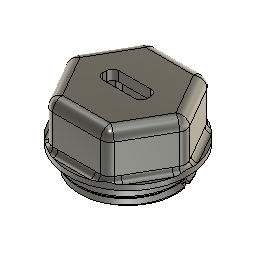
pico_wartel (Autodesk Fusion 360 design; units mm, degrees)
Autodesk Fusion 360 part; units mm, degrees
note: some values were not read from the file. Set by a fixed rule: which sketch regions a step uses.
sketch "Sketch1" plane through (0, 0, 0) normal (0, 0, 1) x (1, 0, 0)
  circle A0 centre (0, 0) radius 10
  constraint coincident A0.centre origin
extrude "Extrude1" add sketch "Sketch1" along normal blind 5
thread "Thread1" "ISO Metric profile 20.0 M20x1.5 6g" major diameter 19.85 minor diameter 18.137 pitch 1.5 angle 60 modelled right hand crest width 0.2154 on face at (9.9876, -0.4985, 3.3333) crest through (9.925, 0, -0.375)
sketch "Sketch2" plane through (0, 0, 5) normal (0, 0, 1) x (-1, 0, 0)
  spline S0 degree 3 poles (5.5723, 8.2131) (4.4831, 8.8876) (3.2736, 9.3446) (0.7674, 9.7621) (-0.5039, 9.7263) (-2.9402, 9.1703) (-4.0834, 8.6632) (-6.0919, 7.248) (-6.9423, 6.3601) (-8.0251, 4.6616) (-8.3649, 3.9377) (-8.8462, 2.4291) (-8.9878, 1.6514) (-9.0271, 0.8652) knots 0 0 0 0 0.384331 0.384331 0.76251 0.76251 1.134533 1.134533 1.5004 1.5004 1.739669 1.739669 1.9762 1.9762 1.9762 1.9762
  arc A0 (-9.0271, 0.8652) -> (-3.7642, -8.2503) centre (0, 0) ccw
  spline S1 degree 3 poles (-3.7642, -8.2503) (-2.7053, -8.7931) (-1.5499, -9.1219) (0.8427, -9.3239) (2.0575, -9.1871) (4.3877, -8.453) (5.4781, -7.8552) (7.3873, -6.2646) (8.1826, -5.2812) (9.1631, -3.4286) (9.4586, -2.6354) (9.8416, -0.9842) (9.9252, -0.1326) (9.8989, 0.7191) knots 0 0 0 0 0.356967 0.356967 0.720082 0.720082 1.089343 1.089343 1.464748 1.464748 1.717242 1.717242 1.972467 1.972467 1.972467 1.972467
  arc A1 (9.8989, 0.7191) -> (5.5723, 8.2131) centre (0, 0) ccw
  circle A2 centre (0, 0) radius 12
  dimension "d3" = 24
  constraint concentric A0 A2
  measures "d3" diameter of A2
extrude "Extrude2" add sketch "Sketch2" along normal blind 1 contours S0 A0 S1 A1 | A2
sketch "Sketch3" plane through (0, 0, 6) normal (0, 0, 1) x (-1, 0, 0)
  circle A0 centre (0, 0) radius 12
  line L0 (-6, -10.3923) -> (6, -10.3923)
  line L1 (6, -10.3923) -> (12, 0)
  line L2 (12, 0) -> (6, 10.3923)
  line L3 (6, 10.3923) -> (-6, 10.3923)
  line L4 (-6, 10.3923) -> (-12, 0)
  line L5 (-12, 0) -> (-6, -10.3923)
  constraint coincident A0.centre origin
  constraint horizontal L0
  constraint coincident A0 L4.end
extrude "Extrude3" add sketch "Sketch3" along normal blind 9 contours L0 L1 L2 L3 L4 L5
sketch "Sketch5" plane through (0, 0, 15) normal (0, 0, 1) x (-1, 0, 0)
  line L0 (-12, 0) -> (-6, -10.3923)
  line L1 (-6, -10.3923) -> (6, -10.3923)
  line L2 (6, -10.3923) -> (12, 0)
  line L3 (12, 0) -> (6, 10.3923)
  line L4 (6, 10.3923) -> (-6, 10.3923)
  line L5 (-6, 10.3923) -> (-12, 0)
  line L6 (-3, 1.625) -> (3.5, 1.625)
  line L7 (4.75, 0.375) -> (4.75, -0.375)
  line L8 (3.5, -1.625) -> (-3, -1.625)
  line L9 (-4.25, -0.375) -> (-4.25, 0.375)
  arc A0 (-3, 1.625) -> (-4.25, 0.375) centre (-3, 0.375) ccw
  arc A1 (-4.25, -0.375) -> (-3, -1.625) centre (-3, -0.375) ccw
  arc A2 (3.5, -1.625) -> (4.75, -0.375) centre (3.5, -0.375) ccw
  arc A3 (4.75, 0.375) -> (3.5, 1.625) centre (3.5, 0.375) ccw
  line L10 (-6, 10.3923) -> (6, -10.3923) construction
  dimension "d40" = 9
  dimension "d41" = 1.25
  dimension "d42" = 3.25
  constraint horizontal L6
  constraint horizontal L8
  constraint vertical L9
  constraint tangent L6 A0
  constraint tangent L9 A0
  constraint tangent L8 A1
  constraint tangent L9 A1
  constraint equal A0 A1
  constraint tangent L7 A2
  constraint tangent L8 A2
  constraint equal A0 A2
  constraint tangent L6 A3
  constraint tangent L7 A3
  constraint equal A0 A3
  constraint coincident L4.end L5.start
  constraint coincident L1.end L2.start
  measures "d40" distance of L7 L9
  measures "d41" radius of A0
  measures "d42" distance of L6 L8
extrude "Extrude5" cut sketch "Sketch5" against normal through all contours L6 L7 L8 L9 A0 A1 A2 A3
sketch "Sketch6" plane through (0, 0, 0) normal (0, 0, -1) x (1, 0, 0)
  line L0 (4.25, 0.375) -> (4.25, -0.375)
  arc A0 (3, -1.625) -> (4.25, -0.375) centre (3, -0.375) ccw
  line L1 (3, -1.625) -> (-3.5, -1.625)
  arc A1 (-4.75, -0.375) -> (-3.5, -1.625) centre (-3.5, -0.375) ccw
  line L2 (-4.75, -0.375) -> (-4.75, 0.375)
  arc A2 (-3.5, 1.625) -> (-4.75, 0.375) centre (-3.5, 0.375) ccw
  line L3 (-3.5, 1.625) -> (3, 1.625)
  arc A3 (4.25, 0.375) -> (3, 1.625) centre (3, 0.375) ccw
  line L4 (-9.25, -1.625) -> (9.25, -1.625)
  line L5 (9.25, -1.625) -> (9.25, -2.875)
  line L6 (9.25, -2.875) -> (-9.25, -2.875)
  line L7 (-9.25, -2.875) -> (-9.25, -1.625)
  line L8 (0, 12.1614) -> (0, -9.8386) construction
  line L9 (-4.75, 0) -> (-4.75, -1.625)
  line L10 (4.25, 0) -> (4.25, -1.625)
  line L11 (5.5, -2.875) -> (-5.5, -2.875)
  line L12 (-5.5, -2.875) -> (-5.5, -4.375)
  line L13 (-5.5, -4.375) -> (5.5, -4.375)
  line L14 (5.5, -4.375) -> (5.5, -2.875)
  line L15 (6.5, -1.625) -> (-6.5, -1.625)
  line L16 (-6.5, -1.625) -> (-6.5, 1.375)
  line L17 (-6.5, 1.375) -> (6.5, 1.375)
  line L18 (6.5, 1.375) -> (6.5, -1.625)
  spline S0 degree 3 poles (-5.2629, 7.3851) (-6.2623, 6.7394) (-7.1248, 5.9032) (-8.4961, 3.9321) (-8.985, 2.8117) (-9.5144, 0.4267) (-9.5419, -0.8166) (-9.119, -3.2653) (-8.6649, -4.4457) (-7.5508, -6.2211) (-7.0116, -6.8737) (-5.7732, -8.031) (-5.0775, -8.5292) (-4.3267, -8.9323) knots 0 0 0 0 0.356967 0.356967 0.720082 0.720082 1.089343 1.089343 1.464748 1.464748 1.717242 1.717242 1.972467 1.972467 1.972467 1.972467
  arc A4 (-4.3267, -8.9323) -> (4.3267, -8.9323) centre (0, 0) ccw
  spline S1 degree 3 poles (4.3267, -8.9323) (5.4554, -8.3263) (6.4559, -7.5074) (8.0706, -5.5456) (8.6752, -4.4268) (9.4118, -2.0389) (9.5442, -0.7953) (9.3229, 1.6517) (8.9791, 2.8322) (8.0496, 4.6191) (7.5926, 5.2754) (6.5267, 6.4465) (5.924, 6.958) (5.2629, 7.3851) knots 0 0 0 0 0.384331 0.384331 0.76251 0.76251 1.134533 1.134533 1.5004 1.5004 1.739669 1.739669 1.9762 1.9762 1.9762 1.9762
  arc A5 (5.2629, 7.3851) -> (-5.2629, 7.3851) centre (0, 0) ccw
  dimension "d15" = 1.25
  dimension "d16" = 18.5
  dimension "d24" = 1.5
  dimension "d25" = 11
  dimension "d26" = 3
  dimension "d27" = 13
  constraint horizontal L4
  constraint vertical L5
  constraint horizontal L6
  constraint vertical L7
  constraint vertical L8
  constraint symmetric L5 L7 L8
  constraint midpoint L2 L9.start
  constraint coincident L4 L9.end
  constraint perpendicular L4 L9
  constraint midpoint L0 L10.start
  constraint coincident L4 L10.end
  constraint perpendicular L4 L10
  constraint collinear L1 L4
  constraint coincident A4.centre L8
  constraint horizontal L11
  constraint vertical L12
  constraint horizontal L13
  constraint vertical L14
  constraint coincident L6 L11.start
  constraint symmetric L8 L12 L14
  constraint horizontal L15
  constraint vertical L16
  constraint horizontal L17
  constraint vertical L18
  constraint coincident L4 L15.start
  measures "d15" distance of L4 L6
  measures "d16" distance of L5 L7
  measures "d24" distance of L11 L13
  measures "d25" distance of L12.end L13.end
  measures "d26" distance of L15.end L16.end
  measures "d27" distance of L16.end L17.end
extrude "Extrude6" cut sketch "Sketch6" against normal up to surface (13 mm away) contours L0 A3 L4 L10 L15 L17 L18 | A0 L4 L10 L15 | L2 A2 L4 L9 L15 L16 L17 | L1 L4 L5 L6 L7 L11 L15 S0 S1 | A1 L4 L9 L15 | L5 L6 S1 | L6 L7 S0 | L6 L11 L12 L13 L14
fillet "Fillet3" radius 2 6 edges at (-9, 5.1962, 15) (0, 10.3923, 15) (9, 5.1962, 15) (9, -5.1962, 15) (0, -10.3923, 15) (-9, -5.1962, 15)
fillet "Fillet3" radius 2 6 edges at (-6, 10.3923, 10.5) (6, 10.3923, 10.5) (12, 0, 10.5) (6, -10.3923, 10.5) (-6, -10.3923, 10.5) (-12, 0, 10.5)
sketch "Sketch8" plane through (0, 0, 0) normal (0, 0, -1) x (1, 0, 0)
  line L0 (3.75, 1.375) -> (6.5, 1.375)
  line L1 (6.5, 1.375) -> (6.5, -1.625)
  line L2 (6.5, -1.625) -> (9.25, -1.625)
  line L3 (9.25, -1.625) -> (9.25, -2.4505)
  line L4 (-9.25, -2.4505) -> (-9.25, -1.625)
  line L5 (-9.25, -1.625) -> (-6.5, -1.625)
  line L6 (-6.5, -1.625) -> (-6.5, 1.375)
  line L7 (-6.5, 1.375) -> (-4.25, 1.375)
  arc A0 (-3.5, 1.625) -> (-4.25, 1.375) centre (-3.5, 0.375) ccw
  line L8 (-3.5, 1.625) -> (3, 1.625)
  arc A1 (3.75, 1.375) -> (3, 1.625) centre (3, 0.375) ccw
  line L9 (-6.5, -1.625) -> (-11.6505, -1.625)
  line L10 (-11.6505, -1.625) -> (-11.6505, -2.875)
  line L11 (-11.6505, -2.875) -> (-6.5, -2.875)
  line L12 (-6.5, -2.875) -> (-6.5, -1.625)
  line L13 (-5.5, -2.875) -> (-9.1467, -2.875)
  circle A2 centre (0, 0) radius 12
  line L14 (6.5, -1.625) -> (11.8895, -1.625)
  line L15 (11.8895, -1.625) -> (11.8895, -2.875)
  line L16 (11.8895, -2.875) -> (6.5, -2.875)
  line L17 (6.5, -2.875) -> (6.5, -1.625)
  line L18 (9.1467, -2.875) -> (5.5, -2.875)
  spline S0 degree 3 poles (9.25, -2.4505) (9.4575, -1.5038) (9.5202, -0.5296) (9.3229, 1.6517) (8.9791, 2.8322) (8.0496, 4.6191) (7.5926, 5.2754) (6.5267, 6.4465) (5.924, 6.958) (5.2629, 7.3851) knots 0.84262 0.84262 0.84262 0.84262 1.134533 1.134533 1.5004 1.5004 1.739669 1.739669 1.9762 1.9762 1.9762 1.9762
  arc A3 (5.2629, 7.3851) -> (-5.2629, 7.3851) centre (0, 0) ccw
  spline S1 degree 3 poles (-5.2629, 7.3851) (-6.2623, 6.7394) (-7.1248, 5.9032) (-8.4961, 3.9321) (-8.985, 2.8117) (-9.5144, 0.4267) (-9.5419, -0.8166) (-9.3079, -2.1715) (-9.2805, -2.3114) (-9.25, -2.4505) knots 0 0 0 0 0.356967 0.356967 0.720082 0.720082 1.089343 1.089343 1.132102 1.132102 1.132102 1.132102
  constraint horizontal L9
  constraint vertical L10
  constraint horizontal L11
  constraint vertical L12
  constraint coincident L5.end L6.start
  constraint collinear L11 L13
  constraint coincident L10.end A2
  constraint horizontal L14
  constraint vertical L15
  constraint horizontal L16
  constraint vertical L17
  constraint coincident L1.end L2.start
  constraint collinear L16 L18
  constraint coincident A2 L14.end
extrude "Extrude7" cut sketch "Sketch8" against normal up to surface (5 mm away) contours L2 L3 A2 L14 L16 L17 L18 S0 | L4 L5 L9 L10 L11 L12 L13 S1
sketch "Sketch9" plane through (0, 0, 0) normal (0, 0, -1) x (1, 0, 0)
  line L0 (3.75, 1.375) -> (6.5, 1.375)
  line L1 (6.5, 1.375) -> (6.5, -1.625)
  line L2 (6.5, -1.625) -> (9.25, -1.625)
  line L3 (9.25, -1.625) -> (9.25, -2.4505)
  line L4 (-9.25, -2.4505) -> (-9.25, -1.625)
  line L5 (-9.25, -1.625) -> (-6.5, -1.625)
  line L6 (-6.5, -1.625) -> (-6.5, 1.375)
  line L7 (-6.5, 1.375) -> (-4.25, 1.375)
  arc A0 (-3.5, 1.625) -> (-4.25, 1.375) centre (-3.5, 0.375) ccw
  line L8 (-3.5, 1.625) -> (3, 1.625)
  arc A1 (3.75, 1.375) -> (3, 1.625) centre (3, 0.375) ccw
  circle A2 centre (0, 6) radius 1.25
  line L9 (0, 13.717) -> (0, 13.3935) construction
  line L10 (0, 13.3935) -> (0, -12.1975) construction
  circle A3 centre (0, -7) radius 1.25
  spline S0 degree 3 poles (9.25, -2.4505) (9.4575, -1.5038) (9.5202, -0.5296) (9.3229, 1.6517) (8.9791, 2.8322) (8.0496, 4.6191) (7.5926, 5.2754) (6.5267, 6.4465) (5.924, 6.958) (5.2629, 7.3851) knots 0.84262 0.84262 0.84262 0.84262 1.134533 1.134533 1.5004 1.5004 1.739669 1.739669 1.9762 1.9762 1.9762 1.9762
  arc A4 (5.2629, 7.3851) -> (-5.2629, 7.3851) centre (0, 0) ccw
  spline S1 degree 3 poles (-5.2629, 7.3851) (-6.2623, 6.7394) (-7.1248, 5.9032) (-8.4961, 3.9321) (-8.985, 2.8117) (-9.4847, 0.5603) (-9.5328, -0.5407) (-9.3933, -1.625) knots 0 0 0 0 0.356967 0.356967 0.720082 0.720082 1.048301 1.048301 1.048301 1.048301
  spline S2 degree 3 poles (-9.3933, -1.625) (-9.3759, -1.7606) (-9.3555, -1.8959) (-9.3079, -2.1715) (-9.2805, -2.3114) (-9.25, -2.4505) knots 1.048301 1.048301 1.048301 1.048301 1.089343 1.089343 1.132102 1.132102 1.132102 1.132102
  dimension "d34" = 2.5
  dimension "d35" = 2.5
  dimension "d36" = 7
  dimension "d37" = 6
  constraint vertical L9
  constraint parallel L9 L10
  constraint coincident L10 A3.centre
  constraint coincident A4.centre L10
  constraint coincident A2.centre L10
  measures "d34" diameter of A2
  measures "d35" diameter of A3
  measures "d36" distance of A4.centre A3.centre
  measures "d37" distance of A4.centre A2.centre
extrude "Extrude8" cut sketch "Sketch9" against normal blind 10 contours A2 | A3
fillet "Fillet4" radius 1 12 edges at (-9, -5.1962, 6) (-11.6906, 0, 6) (-9, 5.1962, 6) (-5.8453, 10.1244, 6) (0, 10.3923, 6) (5.8453, 10.1244, 6) (9, 5.1962, 6) (11.6906, 0, 6) (9, -5.1962, 6) (5.8453, -10.1244, 6) (0, -10.3923, 6) (-5.8453, -10.1244, 6)
sketch "Sketch10" plane through (0, 0, 0) normal (0, 1, 0) x (1, 0, 0)
  line L0 (10, -5) -> (9, -5)
  line L1 (9, -5) -> (9, -4)
  line L2 (9, -4) -> (10, -4)
  line L3 (10, -4) -> (10, -5)
  line L4 (-12, -5) -> (12, -5)
  line L5 (8.25, 0) -> (10, -1)
  line L6 (10, -1) -> (10, 0)
  line L7 (10, 0) -> (8.25, 0)
  dimension "d47" = 9
  dimension "d48" = 10
  dimension "d49" = 1
  dimension "d50" = 8.25
  dimension "d51" = 10
  dimension "d52" = 1
  constraint horizontal L0
  constraint vertical L1
  constraint horizontal L2
  constraint vertical L3
  constraint coincident L0.start L4
  constraint perpendicular L2 L6
  constraint perpendicular L3 L7
  measures "d47" distance of origin L1
  measures "d48" distance of origin L3
  measures "d49" distance of L0.start L2.end
  measures "d50" distance of origin L5.start
  measures "d51" distance of origin L6.end
  measures "d52" distance of L5.end L6.end
revolve "Revolve1" cut sketch "Sketch10" angle 360 about axis through (0, 0, 1.75) along (0, 0, 1)
equation "d35 = d34"
equation "d51 = d48"
